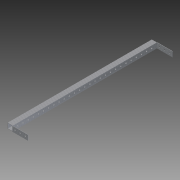
# Autodesk Inventor part: Ridgidizer backbone
Saved by Autodesk Inventor 2012 (Build 160160000, 160)
## iProperties
Created: 2013-05-14
Part Number: Ridgidizer backbone
Material: Default
Document SubType Name: Modeling
Designer: Fabian
Density: 1 g/cm^3
Author: Fabian
Autodesk Inventor part; units mm, degrees
ref_plane "YZ Plane" through (0, 0, 0) normal (1, 0, 0) x (0, 1, 0)
ref_plane "XZ Plane" through (0, 0, 0) normal (0, 1, 0) x (-1, 0, 0)
ref_plane "XY Plane" through (0, 0, 0) normal (0, 0, 1) x (1, 0, 0)
sketch "Sketch1" plane through (0, 0, 0) normal (0, 0, 1) x (1, 0, 0)
  line L0 (-17.8684, 6.9721) -> (7.5316, 6.9721)
  line L1 (7.5316, 6.9721) -> (7.5316, -18.4279)
  line L2 (7.5316, -18.4279) -> (-17.8684, -18.4279)
  line L3 (-17.8684, -18.4279) -> (-17.8684, 6.9721)
  line L4 (-16.2809, 5.3846) -> (5.9441, 5.3846)
  line L5 (5.9441, 5.3846) -> (5.9441, -16.8404)
  line L6 (5.9441, -16.8404) -> (-16.2809, -16.8404)
  line L7 (-16.2809, -16.8404) -> (-16.2809, 5.3846)
  point P0 (0, 0)
  dimension "d0" = 25.4
  dimension "d1" = 25.4
  dimension "d3" = 1.5875
  dimension "d4" = 1.5875
  dimension "d5" = 1.5875
  dimension "d6" = 1.5875
  constraints: 16 end point, 4 parallel, 2 horizontal, 2 perpendicular
  measures "d0" distance of L0.start L0.end
  measures "d1" distance of L2.end L0.start
  measures "d3" distance between parallel lines of L0 L4
  measures "d4" distance between parallel lines of L1 L5
  measures "d5" distance between parallel lines of L2 L6
  measures "d6" distance between parallel lines of L7 L3
extrude "Extrusion1" add sketch "Sketch1" along normal blind 711.2
sketch "Sketch2" plane through (7.5316, -18.4279, 0) normal (1, 0, 0) x (0, 0, -1)
  line L0 (0, 25.4) -> (1.5875, 25.4)
  line L1 (1.5875, 25.4) -> (1.5875, 0)
  line L2 (1.5875, 0) -> (0, 0)
  line L3 (0, 0) -> (0, 25.4)
  line L4 (-711.2, 25.4) -> (-712.7875, 25.4)
  line L5 (-712.7875, 25.4) -> (-712.7875, 0)
  line L6 (-712.7875, 0) -> (-711.2, 0)
  line L7 (-711.2, 0) -> (-711.2, 25.4)
  point P0 (0, 18.4279)
  dimension "d9" = 1.5875
  dimension "d10" = 1.5875
  constraints: 16 end point, 4 parallel, 2 horizontal, 2 perpendicular
  measures "d9" distance between parallel lines of L7 L5
  measures "d10" distance of L0.start L0.end
extrude "Extrusion2" add sketch "Sketch2" along normal blind 76.2
sketch "Sketch3" plane through (-17.8684, -18.4279, 0) normal (-1, 0, 0) x (0, 0, 1)
  line L0 (0, 25.4) -> (711.2, 25.4) projected
  line L1 (0, 0) -> (0, 25.4) projected
  line L2 (0, 0) -> (711.2, 0) projected
  point P0 (0, 18.4279)
  point P1 (25.4, 12.7)
  point P2 (50.8, 12.7)
  point P3 (76.2, 12.7)
  point P4 (101.6, 12.7)
  point P5 (127, 12.7)
  point P6 (152.4, 12.7)
  point P7 (177.8, 12.7)
  point P8 (203.2, 12.7)
  point P9 (228.6, 12.7)
  point P10 (254, 12.7)
  point P11 (279.4, 12.7)
  point P12 (304.8, 12.7)
  point P13 (330.2, 12.7)
  point P14 (355.6, 12.7)
  point P15 (381, 12.7)
  point P16 (406.4, 12.7)
  point P17 (431.8, 12.7)
  point P18 (457.2, 12.7)
  point P19 (482.6, 12.7)
  point P20 (508, 12.7)
  point P21 (533.4, 12.7)
  point P22 (558.8, 12.7)
  point P23 (584.2, 12.7)
  point P24 (609.6, 12.7)
  point P25 (635, 12.7)
  point P26 (660.4, 12.7)
  point P27 (685.8, 12.7)
  dimension "d13" = 25.4
  dimension "d14" = 12.7
  dimension "d17" = 25.4
  constraints: 1 horizontal, 26 other
  measures "d13" distance from line of L1 point (25.4, 12.7)
  measures "d14" distance from line of L2 point (25.4, 12.7)
  measures "d17" distance of point (25.4, 12.7) point (50.8, 12.7)
hole "Hole1" at (-17.8684, -5.7279, 25.4) at (-17.8684, -5.7279, 50.8) at (-17.8684, -5.7279, 76.2) at (-17.8684, -5.7279, 101.6) at (-17.8684, -5.7279, 127) at (-17.8684, -5.7279, 152.4) at (-17.8684, -5.7279, 177.8) at (-17.8684, -5.7279, 203.2) at (-17.8684, -5.7279, 228.6) at (-17.8684, -5.7279, 254) at (-17.8684, -5.7279, 279.4) at (-17.8684, -5.7279, 304.8) at (-17.8684, -5.7279, 330.2) at (-17.8684, -5.7279, 355.6) at (-17.8684, -5.7279, 381) at (-17.8684, -5.7279, 406.4) at (-17.8684, -5.7279, 431.8) at (-17.8684, -5.7279, 457.2) at (-17.8684, -5.7279, 482.6) at (-17.8684, -5.7279, 508) at (-17.8684, -5.7279, 533.4) at (-17.8684, -5.7279, 558.8) at (-17.8684, -5.7279, 584.2) at (-17.8684, -5.7279, 609.6) at (-17.8684, -5.7279, 635) at (-17.8684, -5.7279, 660.4) at (-17.8684, -5.7279, 685.8) direction (1, 0, 0) diameter 6.35 end through all
sketch "Sketch4" plane through (7.5316, -18.4279, 712.7875) normal (0, 0, 1) x (1, 0, 0)
  line L0 (0, 25.4) -> (76.2, 25.4) projected
  line L1 (0, 25.4) -> (0, 0) projected
  point P0 (-7.5316, 18.4279)
  point P1 (12.7, 12.7)
  point P2 (63.5, 12.7)
  point P3 (38.1, 12.7)
  dimension "d29" = 12.7
  dimension "d30" = 12.7
  dimension "d31" = 12.7
  dimension "d32" = 12.7
  dimension "d33" = 25.4
  dimension "d34" = 25.4
  measures "d29" distance from line of L0 point (12.7, 12.7)
  measures "d30" distance from line of L0 point (38.1, 12.7)
  measures "d31" distance from line of L0 point (63.5, 12.7)
  measures "d32" distance from line of L1 point (12.7, 12.7)
  measures "d33" distance of point (38.1, 12.7) point (12.7, 12.7)
  measures "d34" distance of point (63.5, 12.7) point (38.1, 12.7)
hole "Hole2" at (20.2316, -5.7279, 712.7875) at (71.0316, -5.7279, 712.7875) at (45.6316, -5.7279, 712.7875) direction (0, 0, -1) diameter 6.35 end through all
equation "\"d1\" = d0"
equation "\"d4\" = d3"
equation "\"d5\" = d3"
equation "\"d6\" = d3"
body "Solid1"
